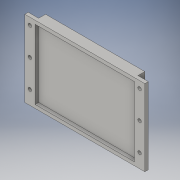
# Autodesk Inventor part: TallFrontWall
Saved by Autodesk Inventor 2016 (Build 200138000, 138)
## iProperties
Created: 2017-01-04
Part Number: TallFrontWall
Material: Generic
Document SubType Name: Modeling
Designer: james
Density: 1 g/cm^3
Appearance: Default
Author: james
Autodesk Inventor part; units mm, degrees
ref_plane "YZ Plane" through (0, 0, 0) normal (1, 0, 0) x (0, 1, 0)
ref_plane "XZ Plane" through (0, 0, 0) normal (0, 1, 0) x (-1, 0, 0)
ref_plane "XY Plane" through (0, 0, 0) normal (0, 0, 1) x (1, 0, 0)
sketch "Sketch1" plane through (0, 0, 0) normal (0, 1, 0) x (-1, 0, 0)
  line L0 (107.2514, 61.1758) -> (-112.4586, 61.1758)
  line L1 (-112.4586, 61.1758) -> (-112.4586, 42.1258)
  line L2 (-112.4586, 42.1258) -> (107.2514, 42.1258)
  line L3 (107.2514, 42.1258) -> (107.2514, 61.1758)
  point P0 (0, 0)
  dimension "d0" = 219.71
  dimension "d1" = 19.05
  constraints: 8 end point, 2 parallel, 1 horizontal, 1 perpendicular
  measures "d0" distance of L1.end L2.end
  measures "d1" distance of L2.end L0.start
extrude "Extrusion1" add sketch "Sketch1" along normal blind 139.7
sketch "Sketch2" plane through (-107.2514, 0, 61.1758) normal (0, 0, 1) x (1, 0, 0)
  line L0 (0, 0) -> (219.71, 0) projected
  line L1 (0, 139.7) -> (219.71, 139.7) projected
  line L2 (0, 0) -> (0, 139.7) projected
  line L3 (219.71, 0) -> (219.71, 139.7) projected
  point P0 (107.2514, 0)
  point P1 (9.525, 76.2)
  point P2 (9.525, 25.4)
  point P3 (210.185, 25.4)
  point P4 (210.185, 76.2)
  dimension "d4" = 0
  dimension "d5" = 0
  dimension "d6" = 0
  dimension "d7" = 0
  dimension "d8" = 25.4
  dimension "d10" = 9.525
  dimension "d11" = 9.525
  dimension "d57" = 50.8
  measures "d4" vertical distance of point (9.525, 76.2) point (210.185, 76.2)
  measures "d5" horizontal distance of point (9.525, 25.4) point (9.525, 76.2)
  measures "d6" horizontal distance of point (210.185, 25.4) point (210.185, 76.2)
  measures "d7" vertical distance of point (9.525, 25.4) point (210.185, 25.4)
  measures "d8" distance from line of L0 point (9.525, 25.4)
  measures "d10" distance from line of L2 point (9.525, 76.2)
  measures "d11" distance from line of L3 point (210.185, 25.4)
  measures "d57" distance of point (9.525, 25.4) point (9.525, 76.2)
hole "Hole1" at (-97.7264, 76.2, 61.1758) at (-97.7264, 25.4, 61.1758) at (102.9336, 25.4, 61.1758) at (102.9336, 76.2, 61.1758) direction (0, 0, -1) diameter 6.35 end through all
sketch "Sketch3" plane through (-107.2514, 0, 61.1758) normal (0, 0, 1) x (1, 0, 0)
  line L0 (19.05, 133.35) -> (200.66, 133.35)
  line L1 (200.66, 133.35) -> (200.66, 6.35)
  line L2 (200.66, 6.35) -> (19.05, 6.35)
  line L3 (19.05, 6.35) -> (19.05, 133.35)
  line L4 (0, 0) -> (0, 139.7) projected
  line L5 (219.71, 0) -> (219.71, 139.7) projected
  line L6 (219.71, 139.7) -> (0, 139.7) projected
  line L7 (0, 0) -> (219.71, 0) projected
  point P0 (107.2514, 0)
  dimension "d19" = 19.05
  dimension "d20" = 19.05
  dimension "d21" = 6.35
  dimension "d22" = 6.35
  constraints: 8 end point, 2 parallel, 1 horizontal, 1 perpendicular
  measures "d19" distance between parallel lines of L4 L3
  measures "d20" distance between parallel lines of L5 L1
  measures "d21" distance between parallel lines of L6 L0
  measures "d22" distance between parallel lines of L7 L2
extrude "Extrusion2" cut sketch "Sketch3" against normal blind 6.35 contours L0 L1 L2 L3
sketch "Sketch6" plane through (0, 139.7, 0) normal (0, 1, 0) x (1, 0, 0)
  line L0 (-88.2014, -54.8258) -> (-107.2514, -54.8258)
  line L1 (-107.2514, -54.8258) -> (-107.2514, -42.1258)
  line L2 (-107.2514, -42.1258) -> (-88.2014, -42.1258)
  line L3 (-88.2014, -42.1258) -> (-88.2014, -54.8258)
  line L4 (112.4586, -42.1258) -> (-107.2514, -42.1258) projected
  line L5 (-107.2514, -42.1258) -> (-107.2514, -61.1758) projected
  line L6 (112.4586, -54.8258) -> (93.4086, -54.8258)
  line L7 (93.4086, -54.8258) -> (93.4086, -42.1258)
  line L8 (93.4086, -42.1258) -> (112.4586, -42.1258)
  line L9 (112.4586, -42.1258) -> (112.4586, -54.8258)
  line L10 (112.4586, -61.1758) -> (112.4586, -42.1258) projected
  line L11 (-107.2514, -61.1758) -> (112.4586, -61.1758) projected
  point P0 (0, 0)
  dimension "d25" = 0
  dimension "d26" = 12.7
  dimension "d27" = 0
  dimension "d28" = 19.05
  dimension "d32" = 19.05
  dimension "d33" = 0
  dimension "d34" = 6.35
  constraints: 16 end point, 4 parallel, 2 horizontal, 2 perpendicular, 1 point on line
  measures "d25" distance between parallel lines of L4 L2
  measures "d26" distance between parallel lines of L2 L0
  measures "d27" distance between parallel lines of L1 L5
  measures "d28" distance between parallel lines of L1 L3
  measures "d32" distance between parallel lines of L7 L9
  measures "d33" distance between parallel lines of L9 L10
  measures "d34" distance between parallel lines of L11 L6
extrude "Extrusion3" cut sketch "Sketch6" against normal blind 254 contours L0 L1 L2 L3 | L4 L9 L6 L7
sketch "Sketch7" plane through (0, 0, 0) normal (0, -1, 0) x (1, 0, 0)
  line L0 (112.4586, 61.1758) -> (112.4586, 42.1258) projected
  line L1 (112.4586, 42.1258) -> (-107.2514, 42.1258) projected
  line L2 (-107.2514, 42.1258) -> (-107.2514, 61.1758) projected
  point P0 (0, 0)
  point P1 (61.6586, 51.6508)
  point P2 (-56.4514, 51.6508)
  point P3 (112.4586, 54.8258)
  point P4 (93.4086, 42.1258)
  point P5 (-88.2014, 42.1258)
  point P6 (-107.2514, 54.8258)
  dimension "d37" = 50.8
  dimension "d38" = 9.525
  dimension "d39" = 50.8
  dimension "d40" = 9.525
  measures "d37" distance from line of point (61.659, 51.651) L0
  measures "d38" distance from line of point (61.659, 51.651) L1
  measures "d39" distance from line of L2 point (-56.451, 51.651)
  measures "d40" distance from line of L1 point (-56.451, 51.651)
hole "Hole2" at (61.6586, 0, 51.6508) at (-56.4514, 0, 51.6508) direction (0, 1, 0) diameter 4.9149 depth 25.4 tip angle 118
sketch "Sketch8" plane through (0, 0, 0) normal (0, -1, 0) x (1, 0, 0)
  line L0 (112.4586, 61.1758) -> (112.4586, 42.1258) projected
  line L1 (112.4586, 42.1258) -> (-107.2514, 42.1258) projected
  point P0 (0, 0)
  point P1 (-1.8414, 51.6508)
  point P2 (-1.8414, 51.6508)
  point P3 (112.4586, 54.8258)
  point P4 (93.4086, 42.1258)
  point P5 (-88.2014, 42.1258)
  dimension "d48" = 114.3
  dimension "d49" = 9.525
  constraints: 1 coincident
  measures "d48" distance from line of L0 point (-1.841, 51.651)
  measures "d49" distance from line of L1 point (-1.841, 51.651)
hole "Hole3" at (-1.8414, 0, 51.6508) direction (0, 1, 0) diameter 4.9149 depth 25.4 tip angle 118
sketch "Sketch9" plane through (-107.2514, 0, 61.1758) normal (0, 0, 1) x (1, 0, 0)
  circle A0 centre (210.185, 76.2) radius 3.175 projected
  line L0 (219.71, 0) -> (219.71, 139.7) projected
  line L1 (0, 0) -> (0, 139.7) projected
  point P0 (107.2514, 0)
  point P1 (9.525, 127)
  point P2 (210.185, 127)
  dimension "d58" = 0
  dimension "d59" = 50.8
  dimension "d60" = 9.525
  dimension "d61" = 9.525
  measures "d58" vertical distance of point (210.185, 127) point (9.525, 127)
  measures "d59" distance of A0.centre point (210.185, 127)
  measures "d60" distance from line of L0 point (210.185, 127)
  measures "d61" distance from line of L1 point (9.525, 127)
hole "Hole4" at (-97.7264, 127, 61.1758) at (102.9336, 127, 61.1758) direction (0, 0, -1) diameter 6.35 depth 25.4 tip angle 118
body "Solid1"
